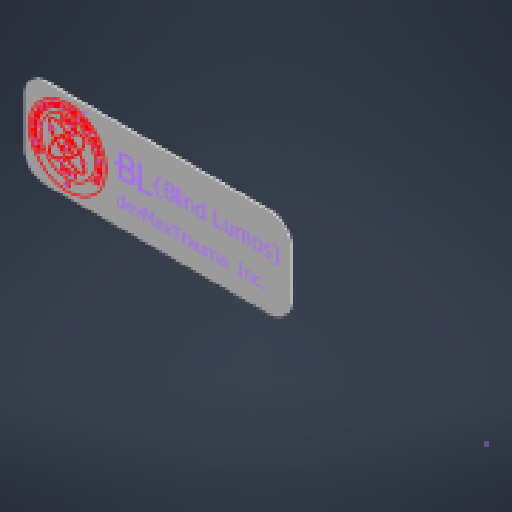
# Autodesk Inventor part: hanabi plate
Saved by Autodesk Inventor 2025.1 (Build 291241020, 241B)
## iProperties
Created: 2024-09-23
Part Number: hanabi plate
Material: Generic
Document SubType Name: Modeling
Designer: techn
Density: 1 g/cm^3
Appearance: Default
Author: techn
Autodesk Inventor part; units mm, degrees
ref_plane "YZ Plane" through (0, 0, 0) normal (1, 0, 0) x (0, 1, 0)
ref_plane "XZ Plane" through (0, 0, 0) normal (0, 1, 0) x (-1, 0, 0)
ref_plane "XY Plane" through (0, 0, 0) normal (0, 0, 1) x (1, 0, 0)
sketch "Sketch1" plane through (0, 0, 0) normal (0, 0, 1) x (1, 0, 0)
  line L0 (3, 0) -> (447, 0)
  line L1 (450, 3) -> (450, 147)
  line L2 (447, 150) -> (3, 150)
  line L3 (0, 147) -> (0, 3)
  arc A0 (3, 150) -> (0, 147) centre (3, 147) ccw
  arc A1 (450, 147) -> (447, 150) centre (447, 147) ccw
  arc A2 (447, 0) -> (450, 3) centre (447, 3) ccw
  arc A3 (0, 3) -> (3, 0) centre (3, 3) ccw
  point P0 (0, 0)
  point P1 (0, 150)
  point P2 (450, 150)
  point P3 (450, 0)
  point P4 (0, 0)
  dimension "d0" = 450
  dimension "d1" = 150
  dimension "d6" = 3
  constraints: 10 point on line, 8 end point, 8 point on circle, 8 tangent, 4 centre point, 3 equal radius, 2 parallel, 1 horizontal, 1 perpendicular
  measures "d0" distance of point (0, 150) point (450, 150)
  measures "d1" distance of point (450, 150) point (450, 0)
  measures "d6" radius of A0
extrude "Extrusion1" add sketch "Sketch1" along normal blind 3
sketch "Sketch2" plane through (0, 0, 3) normal (0, 0, 1) x (1, 0, 0)
  circle A0 centre (74.3304, 73.386) radius 64.4941
  circle A1 centre (74.1358, 19.1374) radius 3.759
  circle A2 centre (74.3304, 73.386) radius 46.1652
  arc A3 (60.0832, 47.8007) -> (66.8292, 50.9644) centre (63.3353, 49.6403) ccw
  arc A4 (102.5659, 60.1821) -> (99.6639, 66.6182) centre (100.186, 62.9813) ccw
  arc A5 (80.1151, 97.5331) -> (86.506, 100.628) centre (82.7963, 100.1425) ccw
  arc A6 (44.8092, 88.9664) -> (47.8294, 82.593) centre (47.2318, 86.2121) ccw
  line L0 (73.0471, 70.515) -> (72.9845, 77.892)
  line L1 (72.9845, 77.892) -> (69.4651, 77.9045)
  line L2 (69.4651, 77.9045) -> (69.5403, 70.4023)
  line L3 (69.5403, 70.4023) -> (62.2134, 70.4148)
  line L4 (62.2134, 70.4148) -> (62.2385, 67.2712)
  line L5 (62.2385, 67.2712) -> (84.0562, 67.2712)
  line L6 (84.0562, 67.2712) -> (84.0562, 70.3898)
  line L7 (84.0562, 70.3898) -> (73.0471, 70.515)
  line L8 (81.7131, 85.3553) -> (64.4794, 85.3954)
  line L9 (64.4794, 85.3954) -> (64.4794, 82.4296)
  line L10 (64.4794, 82.4296) -> (77.8656, 82.4096)
  arc A7 (80.1926, 72.9483) -> (81.7131, 85.3553) centre (16.1968, 87.088) ccw
  arc A8 (76.6977, 73.1086) -> (77.8656, 82.4096) centre (28.8399, 83.8415) ccw
  line L11 (76.6977, 73.1086) -> (80.1926, 72.9483)
  line L12 (22.8218, 44.3119) -> (29.3747, 47.7587)
  line L13 (29.3747, 47.7587) -> (28.6132, 49.3017)
  line L14 (28.6132, 49.3017) -> (25.0462, 47.5182)
  line L15 (25.0462, 47.5182) -> (27.6313, 51.3056)
  line L16 (27.6313, 51.3056) -> (26.8297, 52.8286)
  line L17 (26.8297, 52.8286) -> (20.1165, 49.4821)
  line L18 (20.1165, 49.4821) -> (20.9582, 47.8188)
  line L19 (20.9582, 47.8188) -> (24.3248, 49.5221)
  line L20 (24.3248, 49.5221) -> (21.9, 45.895)
  line L21 (21.9, 45.895) -> (22.8218, 44.3119)
  arc A9 (20.5574, 56.2553) -> (21.4191, 53.8706) centre (21.1012, 55.1038) ccw
  arc A10 (23.0824, 54.552) -> (22.2407, 56.7763) centre (22.685, 55.673) ccw
  arc A11 (21.4191, 53.8706) -> (23.0824, 54.552) centre (20.078, 59.5153) ccw
  arc A12 (24.3636, 53.0797) -> (21.518, 58.5304) centre (22.6001, 55.6272) ccw
  arc A13 (22.1192, 52.1379) -> (24.3636, 53.0797) centre (20.1363, 60.0082) ccw
  line L22 (19.9149, 57.9493) -> (20.5574, 56.2553)
  line L23 (21.518, 58.5304) -> (22.2407, 56.7763)
  line L24 (15.5802, 64.2799) -> (16.032, 62.5112)
  line L25 (16.032, 62.5112) -> (18.4166, 62.9721)
  line L26 (18.4166, 62.9721) -> (18.9176, 61.0684)
  line L27 (18.9176, 61.0684) -> (16.4127, 60.6075)
  line L28 (16.4127, 60.6075) -> (16.8536, 58.7639)
  line L29 (16.8536, 58.7639) -> (24.0877, 60.2668)
  line L30 (24.0877, 60.2668) -> (23.727, 62.0503)
  line L31 (23.727, 62.0503) -> (20.6811, 61.4892)
  line L32 (20.6811, 61.4892) -> (20.3604, 63.3729)
  line L33 (20.3604, 63.3729) -> (23.2661, 64.0342)
  line L34 (23.2661, 64.0342) -> (22.8854, 65.8177)
  line L35 (22.8854, 65.8177) -> (15.5802, 64.2799)
  line L36 (14.9282, 71.5177) -> (15.4291, 66.3877)
  line L37 (15.4291, 66.3877) -> (22.8036, 66.9087)
  line L38 (22.8036, 66.9087) -> (22.3627, 72.3593)
  line L39 (22.3627, 72.3593) -> (20.5191, 72.2191)
  line L40 (20.5191, 72.2191) -> (20.8397, 68.6721)
  line L41 (20.8397, 68.6721) -> (19.6374, 68.632)
  line L42 (19.6374, 68.632) -> (19.4169, 71.5979)
  line L43 (19.4169, 71.5979) -> (17.6334, 71.4776)
  line L44 (17.6334, 71.4776) -> (17.8739, 68.4717)
  line L45 (17.8739, 68.4717) -> (16.9922, 68.4317)
  line L46 (16.9922, 68.4317) -> (16.6716, 71.678)
  line L47 (16.6716, 71.678) -> (14.9282, 71.5177)
  ellipse E0 centre (18.7456, 76.2269) end of major axis (16.6515, 76.3071) minor radius 1.427
  ellipse E1 centre (18.7256, 76.1868) end of major axis (14.828, 76.3872) minor radius 3.5212
  line L48 (15.4067, 81.6515) -> (15.7474, 83.3549)
  line L49 (15.7474, 83.3549) -> (19.8153, 84.6975)
  line L50 (19.8153, 84.6975) -> (16.088, 85.4389)
  line L51 (16.088, 85.4389) -> (16.2884, 87.1623)
  line L52 (16.2884, 87.1623) -> (23.7029, 85.8598)
  line L53 (23.7029, 85.8598) -> (23.5025, 84.2566)
  line L54 (23.5025, 84.2566) -> (19.0338, 82.8138)
  line L55 (19.0338, 82.8138) -> (23.0216, 82.0723)
  line L56 (23.0216, 82.0723) -> (22.7811, 80.2488)
  line L57 (22.7811, 80.2488) -> (15.4067, 81.6515)
  line L58 (19.7752, 97.1418) -> (17.8715, 92.2723)
  line L59 (17.8715, 92.2723) -> (24.745, 89.7073)
  line L60 (24.745, 89.7073) -> (26.6487, 94.6169)
  line L61 (26.6487, 94.6169) -> (25.1658, 95.2581)
  line L62 (25.1658, 95.2581) -> (23.9434, 92.0719)
  line L63 (23.9434, 92.0719) -> (22.6609, 92.5529)
  line L64 (22.6609, 92.5529) -> (23.743, 95.3183)
  line L65 (23.743, 95.3183) -> (22.1599, 95.9395)
  line L66 (22.1599, 95.9395) -> (21.0778, 93.0939)
  line L67 (21.0778, 93.0939) -> (20.0758, 93.4747)
  line L68 (20.0758, 93.4747) -> (21.2782, 96.5206)
  line L69 (21.2782, 96.5206) -> (19.7752, 97.1418)
  line L70 (21.3984, 100.3882) -> (20.3764, 98.765)
  line L71 (20.3764, 98.765) -> (27.0094, 95.3383)
  line L72 (27.0094, 95.3383) -> (29.3339, 99.9273)
  line L73 (29.3339, 99.9273) -> (27.7909, 100.6888)
  line L74 (27.7909, 100.6888) -> (26.3681, 97.8833)
  line L75 (26.3681, 97.8833) -> (21.3984, 100.3882)
  line L76 (29.7347, 100.3882) -> (32.7206, 104.917)
  line L77 (32.7206, 104.917) -> (31.2577, 105.9591)
  line L78 (31.2577, 105.9591) -> (29.2939, 103.0334)
  line L79 (29.2939, 103.0334) -> (28.2518, 103.6746)
  line L80 (28.2518, 103.6746) -> (29.9752, 106.2998)
  line L81 (29.9752, 106.2998) -> (28.5725, 107.1815)
  line L82 (28.5725, 107.1815) -> (26.789, 104.6365)
  line L83 (26.789, 104.6365) -> (25.9674, 105.1976)
  line L84 (25.9674, 105.1976) -> (27.9312, 107.943)
  line L85 (27.9312, 107.943) -> (26.4884, 108.9249)
  line L86 (26.4884, 108.9249) -> (23.4625, 104.6165)
  line L87 (23.4625, 104.6165) -> (29.7347, 100.3882)
  line L88 (32.42, 111.7103) -> (33.6223, 113.073)
  line L89 (34.8848, 112.0109) -> (33.6223, 110.6082)
  arc A14 (30.5404, 107.4866) -> (34.8848, 112.0109) centre (32.7697, 109.6939) ccw
  arc A15 (33.6223, 113.073) -> (29.2378, 108.8017) centre (31.6861, 110.6746) ccw
  arc A16 (29.2378, 108.8017) -> (30.5404, 107.4866) centre (52.0371, 130.0812) ccw
  arc A17 (32.42, 111.7103) -> (30.7157, 109.9915) centre (31.6602, 110.7594) ccw
  arc A18 (32.0912, 108.6533) -> (33.6223, 110.6082) centre (32.9043, 109.5936) ccw
  arc A19 (30.7157, 109.9915) -> (32.0912, 108.6533) centre (34.3325, 112.3331) ccw
  line L90 (36.7024, 119.6663) -> (37.8847, 118.4238)
  line L91 (37.8847, 118.4238) -> (36.502, 117.1413)
  line L92 (36.502, 117.1413) -> (40.2293, 112.913)
  line L93 (40.2293, 112.913) -> (38.8666, 111.6506)
  line L94 (38.8666, 111.6506) -> (35.0391, 115.8588)
  line L95 (35.0391, 115.8588) -> (33.5362, 114.5563)
  line L96 (33.5362, 114.5563) -> (32.3739, 115.8588)
  line L97 (32.3739, 115.8588) -> (36.7024, 119.6663)
  line L98 (38.0651, 120.7283) -> (42.2533, 114.6565)
  line L99 (42.2533, 114.6565) -> (43.636, 115.6584)
  line L100 (43.636, 115.6584) -> (42.2332, 117.8026)
  line L101 (42.2332, 117.8026) -> (43.5558, 118.7044)
  line L102 (38.0651, 120.7283) -> (41.2914, 122.9527)
  line L103 (45.4555, 116.9645) -> (47.0226, 118.023)
  line L104 (47.0226, 118.023) -> (46.7462, 118.4132)
  line L105 (46.7462, 118.4132) -> (46.3989, 118.4328)
  line L106 (46.3989, 118.4328) -> (45.4247, 119.8307)
  line L107 (45.4555, 116.9645) -> (44.134, 118.5977)
  arc A20 (44.134, 118.5977) -> (43.5558, 118.7044) centre (43.8033, 118.4259) ccw
  arc A21 (45.4247, 119.8307) -> (44.2896, 120.3317) centre (44.5184, 119.3138) ccw
  arc A22 (44.2896, 120.3317) -> (41.2914, 122.9527) centre (42.2418, 121.0145) ccw
  line L108 (40.5088, 120.363) -> (41.2524, 119.2828)
  line L109 (41.2524, 119.2828) -> (42.5988, 120.2221)
  line L110 (41.8787, 121.3102) -> (40.5088, 120.363)
  arc A23 (42.5988, 120.2221) -> (41.8787, 121.3102) centre (42.1607, 120.7145) ccw
  ellipse E2 centre (48.8933, 123.1148) end of major axis (47.8713, 124.9484) minor radius 1.3869
  ellipse E3 centre (48.9333, 123.1048) end of major axis (47.0296, 126.4514) minor radius 3.3442
  line L111 (51.8591, 128.6156) -> (53.5824, 129.1767)
  line L112 (53.5824, 129.1767) -> (56.949, 126.3311)
  line L113 (56.949, 126.3311) -> (55.6465, 130.0384)
  line L114 (55.6465, 130.0384) -> (57.2296, 130.4392)
  line L115 (57.2296, 130.4392) -> (59.7144, 123.5256)
  line L116 (59.7144, 123.5256) -> (58.0913, 122.9645)
  line L117 (58.0913, 122.9645) -> (54.6846, 126.0305)
  line L118 (54.6846, 126.0305) -> (55.927, 122.2231)
  line L119 (55.927, 122.2231) -> (54.2838, 121.682)
  line L120 (54.2838, 121.682) -> (51.8591, 128.6156)
  line L121 (59.1333, 130.9602) -> (60.9769, 131.381)
  line L122 (60.9769, 131.381) -> (62.7003, 124.2671)
  line L123 (62.7003, 124.2671) -> (60.9969, 123.8262)
  line L124 (60.9969, 123.8262) -> (59.1333, 130.9602)
  arc A24 (65.2629, 127.4613) -> (67.7678, 127.9022) centre (66.5191, 127.6602) ccw
  arc A25 (67.4947, 129.7232) -> (65.0149, 129.2974) centre (66.2808, 129.3592) ccw
  arc A26 (69.2357, 129.9737) -> (63.1362, 128.9091) centre (66.2187, 129.2539) ccw
  arc A27 (63.4994, 127.1432) -> (69.4235, 128.0199) centre (66.453, 127.6388) ccw
  arc A28 (63.1362, 128.9091) -> (63.4994, 127.1432) centre (67.9042, 128.9695) ccw
  arc A29 (65.0149, 129.2974) -> (65.2629, 127.4613) centre (79.0489, 130.2581) ccw
  line L125 (67.4947, 129.7232) -> (69.2357, 129.9737)
  line L126 (67.7678, 127.9022) -> (69.4235, 128.0199)
  line L127 (73.8923, 132.8018) -> (76.2469, 132.7391)
  line L128 (76.2469, 132.7391) -> (76.9608, 128.5434)
  line L129 (76.9608, 128.5434) -> (78.2132, 132.5638)
  line L130 (78.2132, 132.5638) -> (80.4802, 132.426)
  line L131 (80.4802, 132.426) -> (80.0543, 125.1994)
  line L132 (80.0543, 125.1994) -> (78.4136, 125.2745)
  line L133 (78.4136, 125.2745) -> (78.6015, 128.08)
  line L134 (78.6015, 128.08) -> (77.612, 125.3998)
  line L135 (77.612, 125.3998) -> (75.9588, 125.4123)
  line L136 (75.9588, 125.4123) -> (75.3576, 128.5309)
  line L137 (75.3576, 128.5309) -> (75.1322, 125.4874)
  line L138 (75.1322, 125.4874) -> (73.4414, 125.6002)
  line L139 (73.4414, 125.6002) -> (73.8923, 132.8018)
  line L140 (81.0939, 125.0491) -> (86.279, 123.997)
  line L141 (86.279, 123.997) -> (86.6046, 125.5751)
  line L142 (86.6046, 125.5751) -> (83.0978, 126.2264)
  line L143 (83.0978, 126.2264) -> (83.3984, 127.6041)
  line L144 (83.3984, 127.6041) -> (86.5044, 127.053)
  line L145 (86.5044, 127.053) -> (86.7925, 128.5935)
  line L146 (86.7925, 128.5935) -> (83.7365, 129.1571)
  line L147 (83.7365, 129.1571) -> (83.8994, 130.2342)
  line L148 (83.8994, 130.2342) -> (87.1682, 129.5579)
  line L149 (87.1682, 129.5579) -> (87.5064, 131.1235)
  line L150 (87.5064, 131.1235) -> (82.4841, 132.163)
  line L151 (82.4841, 132.163) -> (81.0939, 125.0491)
  line L152 (89.2849, 130.6976) -> (90.9757, 130.1841)
  line L153 (90.9757, 130.1841) -> (88.9092, 123.208)
  line L154 (88.9092, 123.208) -> (87.1682, 123.6589)
  line L155 (87.1682, 123.6589) -> (89.2849, 130.6976)
  line L156 (90.9953, 125.1721) -> (92.4983, 124.611)
  line L157 (95.3038, 126.0338) -> (96.8869, 125.3725)
  arc A30 (90.9953, 125.1721) -> (96.1053, 122.8275) centre (93.6122, 124.1346) ccw
  arc A31 (96.8869, 125.3725) -> (91.857, 127.4967) centre (94.3068, 126.2803) ccw
  arc A32 (91.857, 127.4967) -> (93.4401, 124.6311) centre (94.2672, 126.9581) ccw
  arc A33 (96.1053, 122.8275) -> (94.9631, 125.6731) centre (93.9846, 123.6283) ccw
  arc A34 (95.3038, 126.0338) -> (93.5403, 127.176) centre (94.2317, 126.311) ccw
  arc A35 (93.5403, 127.176) -> (93.8409, 126.4146) centre (93.9888, 126.913) ccw
  arc A36 (93.8409, 126.4146) -> (94.9631, 125.6731) centre (103.26, 139.4505) ccw
  line L158 (93.4401, 124.6311) -> (94.4822, 123.8896)
  arc A37 (94.2417, 123.048) -> (94.4822, 123.8896) centre (94.0571, 123.5559) ccw
  arc A38 (92.8059, 123.2884) -> (94.2417, 123.048) centre (93.781, 124.7043) ccw
  arc A39 (92.4983, 124.611) -> (92.8059, 123.2884) centre (93.1362, 124.0623) ccw
  line L159 (100.1226, 124.5633) -> (97.4935, 119.6577)
  line L160 (97.4935, 119.6577) -> (99.0966, 118.7279)
  line L161 (99.0966, 118.7279) -> (101.854, 123.7297)
  line L162 (101.854, 123.7297) -> (103.5854, 122.7999)
  line L163 (103.5854, 122.7999) -> (104.419, 124.1786)
  line L164 (104.419, 124.1786) -> (99.3852, 127.0322)
  line L165 (99.3852, 127.0322) -> (98.4554, 125.5893)
  line L166 (98.4554, 125.5893) -> (100.1226, 124.5633)
  line L167 (101.5053, 117.4294) -> (105.7536, 123.4211)
  line L168 (105.7536, 123.4211) -> (109.9218, 120.4353)
  line L169 (109.9218, 120.4353) -> (108.9399, 119.0125)
  line L170 (108.9399, 119.0125) -> (106.1945, 120.8962)
  line L171 (106.1945, 120.8962) -> (105.6935, 120.1948)
  line L172 (105.6935, 120.1948) -> (108.2185, 118.3512)
  line L173 (108.2185, 118.3512) -> (107.2566, 117.0486)
  line L174 (107.2566, 117.0486) -> (104.6715, 118.752)
  line L175 (104.6715, 118.752) -> (103.9501, 117.73)
  line L176 (103.9501, 117.73) -> (106.7957, 115.6659)
  line L177 (106.7957, 115.6659) -> (105.7136, 114.2832)
  line L178 (105.7136, 114.2832) -> (101.5053, 117.4294)
  line L179 (111.3646, 119.1928) -> (106.3147, 113.7422)
  line L180 (106.3147, 113.7422) -> (107.6774, 112.5498)
  line L181 (107.6774, 112.5498) -> (109.501, 114.5037)
  line L182 (109.501, 114.5037) -> (110.7033, 113.5017)
  line L183 (111.3646, 119.1928) -> (114.1864, 116.6281)
  line L184 (112.7774, 115.5656) -> (111.6374, 116.6713)
  line L185 (111.6374, 116.6713) -> (110.8351, 115.7515)
  line L186 (110.8351, 115.7515) -> (111.8772, 114.7094)
  line L187 (110.6791, 112.9268) -> (109.2764, 111.2235)
  line L188 (109.2764, 111.2235) -> (110.7621, 109.8192)
  line L189 (110.7621, 109.8192) -> (111.13, 110.1949)
  line L190 (111.13, 110.1949) -> (111.0282, 110.5706)
  line L191 (111.0282, 110.5706) -> (112.2729, 111.9014)
  arc A40 (110.6791, 112.9268) -> (110.7033, 113.5017) centre (110.3532, 113.2285) ccw
  arc A41 (112.2729, 111.9014) -> (112.4178, 113.0193) centre (111.1593, 112.6141) ccw
  arc A42 (111.8772, 114.7094) -> (112.7774, 115.5656) centre (112.2379, 115.2315) ccw
  arc A43 (112.4178, 113.0193) -> (114.1864, 116.6281) centre (112.538, 115.1982) ccw
  line L192 (113.3248, 107.0457) -> (119.0961, 111.4343)
  line L193 (119.0961, 111.4343) -> (120.2784, 109.9514)
  line L194 (120.2784, 109.9514) -> (118.2144, 108.4284)
  line L195 (118.2144, 108.4284) -> (119.4368, 106.8052)
  line L196 (119.4368, 106.8052) -> (121.4607, 108.3081)
  line L197 (121.4607, 108.3081) -> (122.623, 106.8052)
  line L198 (122.623, 106.8052) -> (116.6714, 102.3966)
  line L199 (116.6714, 102.3966) -> (115.5893, 103.8594)
  line L200 (115.5893, 103.8594) -> (117.9739, 105.683)
  line L201 (117.9739, 105.683) -> (116.8116, 107.3262)
  line L202 (116.8116, 107.3262) -> (114.3268, 105.5227)
  line L203 (114.3268, 105.5227) -> (113.3248, 107.0457)
  line L204 (117.3727, 101.3545) -> (123.5448, 105.162)
  line L205 (123.5448, 105.162) -> (124.5468, 103.5388)
  line L206 (124.5468, 103.5388) -> (118.2745, 99.7314)
  line L207 (118.2745, 99.7314) -> (117.3727, 101.3545)
  line L208 (123.2155, 95.6967) -> (122.5542, 96.8791)
  line L209 (122.5542, 96.8791) -> (124.0572, 97.6606)
  line L210 (124.0572, 97.6606) -> (125.3998, 94.9553)
  line L211 (125.3998, 94.9553) -> (121.6926, 93.0315)
  line L212 (121.6926, 93.0315) -> (120.9912, 94.4142)
  line L213 (120.9912, 94.4142) -> (121.3118, 94.6948)
  arc A44 (121.9731, 98.0213) -> (123.2155, 95.6967) centre (122.9571, 97.0529) ccw
  arc A45 (124.0271, 99.131) -> (121.9731, 98.0213) centre (124.5431, 95.72) ccw
  arc A46 (125.2044, 96.7012) -> (124.0271, 99.131) centre (124.3539, 97.7892) ccw
  line L214 (125.2044, 96.7012) -> (125.981, 95.0354)
  arc A47 (125.981, 95.0354) -> (122.8498, 100.7216) centre (124.119, 97.7153) ccw
  arc A48 (122.8498, 100.7216) -> (120.1946, 98.8178) centre (124.2192, 96.0082) ccw
  arc A49 (120.1946, 98.8178) -> (121.3118, 94.6948) centre (122.701, 97.2841) ccw
  line L215 (122.0117, 92.1357) -> (128.8731, 94.348)
  line L216 (128.8731, 94.348) -> (129.4823, 92.7128)
  line L217 (129.4823, 92.7128) -> (126.9494, 91.8792)
  line L218 (126.9494, 91.8792) -> (127.7509, 89.6989)
  line L219 (127.7509, 89.6989) -> (130.0595, 90.5005)
  line L220 (130.0595, 90.5005) -> (130.6045, 88.9615)
  line L221 (130.6045, 88.9615) -> (123.6469, 86.7492)
  line L222 (123.6469, 86.7492) -> (123.2622, 88.3523)
  line L223 (123.2622, 88.3523) -> (126.0837, 89.3462)
  line L224 (126.0837, 89.3462) -> (125.5386, 91.3662)
  line L225 (125.5386, 91.3662) -> (122.4606, 90.4684)
  line L226 (122.4606, 90.4684) -> (122.0117, 92.1357)
  line L227 (127.1227, 83.2797) -> (127.2229, 81.6766)
  line L228 (129.7879, 79.7628) -> (129.9758, 78.1847)
  arc A50 (127.1227, 83.2797) -> (126.8547, 77.5109) centre (127.4108, 80.3757) ccw
  arc A51 (129.9758, 78.1847) -> (130.081, 83.6629) centre (129.6354, 80.9314) ccw
  arc A52 (130.081, 83.6629) -> (127.8241, 81.7918) centre (129.9946, 81.4705) ccw
  arc A53 (127.2229, 81.6766) -> (126.2836, 80.5769) centre (127.3612, 80.6074) ccw
  arc A54 (126.2836, 80.5769) -> (126.747, 79.4622) centre (127.8549, 80.5765) ccw
  arc A55 (126.747, 79.4622) -> (127.5486, 79.7252) centre (127.0889, 79.7732) ccw
  arc A56 (127.8241, 81.7918) -> (127.5486, 79.7252) centre (778.3659, -5.9988) ccw
  arc A57 (129.7879, 79.7628) -> (130.2163, 81.8419) centre (129.4879, 80.9083) ccw
  arc A58 (130.2163, 81.8419) -> (129.5775, 81.5037) centre (130.0077, 81.4634) ccw
  arc A59 (129.1642, 78.8861) -> (129.5775, 81.5037) centre (45.9299, 93.3698) ccw
  arc A60 (126.8547, 77.5109) -> (129.1642, 78.8861) centre (127.0095, 79.8778) ccw
  ellipse E4 centre (128.9018, 73.4046) end of major axis (126.7676, 73.4246) minor radius 1.3445 (129.8941, 72.2086) -> (128.0696, 72.1712) ccw
  ellipse E5 centre (128.9118, 73.4747) end of major axis (125.0443, 73.4847) minor radius 3.1768 (129.9327, 70.4097) -> (128.0695, 70.3749) ccw
  line L229 (128.0702, 70.3786) -> (128.0695, 70.3749)
  line L230 (129.8941, 72.2086) -> (129.9327, 70.4097)
  line L231 (128.0702, 72.1711) -> (128.0702, 70.3786)
  line L232 (128.0696, 72.1712) -> (128.0702, 72.1711)
  line L233 (125.2047, 69.6146) -> (132.4362, 68.5719)
  line L234 (132.4362, 68.5719) -> (132.2176, 66.7556)
  line L235 (132.2176, 66.7556) -> (129.5436, 67.0415)
  line L236 (129.5436, 67.0415) -> (129.325, 65.0402)
  line L237 (129.325, 65.0402) -> (131.9653, 64.7039)
  line L238 (131.9653, 64.7039) -> (131.6962, 62.9212)
  line L239 (131.6962, 62.9212) -> (124.2629, 63.9303)
  line L240 (124.2629, 63.9303) -> (124.5488, 65.797)
  line L241 (124.5488, 65.797) -> (127.6937, 65.3766)
  line L242 (127.6937, 65.3766) -> (127.9291, 67.2938)
  line L243 (127.9291, 67.2938) -> (124.8683, 67.6469)
  line L244 (124.8683, 67.6469) -> (125.2047, 69.6146)
  ellipse E6 centre (126.872, 58.825) end of major axis (124.9296, 59.4724) minor radius 1.5069
  ellipse E7 centre (126.8552, 58.7829) end of major axis (123.2647, 60.2292) minor radius 3.2341
  ellipse E8 centre (124.2064, 51.5934) end of major axis (122.3397, 52.4763) minor radius 1.4344
  ellipse E9 centre (124.2989, 51.5682) end of major axis (120.9606, 53.5022) minor radius 3.3298
  line L245 (119.6993, 46.8088) -> (118.0344, 44.1012)
  line L246 (118.0344, 44.1012) -> (116.4703, 45.0598)
  line L247 (116.4703, 45.0598) -> (119.0939, 49.3483)
  line L248 (119.0939, 49.3483) -> (125.5518, 45.6484)
  line L249 (125.5518, 45.6484) -> (124.5092, 44.0003)
  line L250 (124.5092, 44.0003) -> (119.6993, 46.8088)
  arc A61 (66.937, 40.1205) -> (61.7975, 40.0936) centre (64.3667, 40.2125) ccw
  arc A62 (65.6866, 40.3787) -> (62.9748, 40.0633) centre (64.3345, 40.1883) ccw
  arc A63 (65.119, 39.1384) -> (65.6866, 40.3787) centre (64.3203, 40.2539) ccw
  line L251 (61.7975, 40.0936) -> (62.9748, 40.0633)
  line L252 (65.119, 39.1384) -> (61.7256, 35.7606)
  line L253 (61.7256, 35.7606) -> (61.7256, 34.6674)
  line L254 (61.7256, 34.6674) -> (66.8718, 34.6674)
  line L255 (66.8718, 34.6674) -> (66.8718, 35.8783)
  line L256 (66.8718, 35.8783) -> (63.4242, 35.8951)
  line L257 (63.4242, 35.8951) -> (66.2664, 38.6364)
  arc A64 (66.2664, 38.6364) -> (66.937, 40.1205) centre (64.8521, 40.169) ccw
  arc A65 (72.6467, 40.4747) -> (69.7982, 40.4852) centre (71.2209, 40.0648) ccw
  arc A66 (73.971, 40.296) -> (68.3687, 40.4432) centre (71.1599, 39.9911) ccw
  arc A67 (69.8087, 36.7223) -> (72.7413, 37.0376) centre (71.2359, 37.243) ccw
  arc A68 (68.3582, 36.8905) -> (74.0236, 37.2689) centre (71.1847, 37.173) ccw
  line L258 (68.3687, 40.4432) -> (68.3582, 36.8905)
  line L259 (69.8087, 36.7223) -> (69.7982, 40.4852)
  line L260 (72.6467, 40.4747) -> (72.7413, 37.0376)
  line L261 (74.0236, 37.2689) -> (73.971, 40.296)
  line L262 (76.2507, 42.6737) -> (78.9247, 42.6737)
  line L263 (78.9247, 42.6737) -> (78.9247, 34.7358)
  line L264 (78.9247, 34.7358) -> (77.6742, 34.7359)
  line L265 (77.6742, 34.7359) -> (77.6633, 41.6142)
  line L266 (77.6633, 41.6142) -> (76.2528, 41.6191)
  line L267 (76.2528, 41.6191) -> (76.2507, 42.6737)
  arc A69 (86.5806, 40.4747) -> (83.7321, 40.4852) centre (85.1548, 40.0648) ccw
  arc A70 (87.905, 40.296) -> (82.3026, 40.4432) centre (85.0938, 39.9911) ccw
  arc A71 (83.7426, 36.7223) -> (86.6752, 37.0376) centre (85.1699, 37.243) ccw
  arc A72 (82.2921, 36.8905) -> (87.9575, 37.2689) centre (85.1186, 37.173) ccw
  line L268 (82.3026, 40.4432) -> (82.2921, 36.8905)
  line L269 (83.7426, 36.7223) -> (83.7321, 40.4852)
  line L270 (86.5806, 40.4747) -> (86.6752, 37.0376)
  line L271 (87.9575, 37.2689) -> (87.905, 40.296)
  line L272 (62.4142, 114.1934) -> (65.0882, 114.1934)
  line L273 (65.0882, 114.1934) -> (65.0882, 106.2555)
  line L274 (65.0882, 106.2555) -> (63.8378, 106.2556)
  line L275 (63.8378, 106.2556) -> (63.8269, 113.1339)
  line L276 (63.8269, 113.1339) -> (62.4164, 113.1388)
  line L277 (62.4164, 113.1388) -> (62.4142, 114.1934)
  circle A73 centre (71.262, 111.5976) radius 1.6109
  arc A74 (73.6726, 110.1228) -> (71.3999, 108.7522) centre (71.2213, 111.6179) ccw
  line L278 (69.6746, 106.3394) -> (71.2772, 106.3522)
  line L279 (71.2772, 106.3522) -> (73.6726, 110.1228)
  line L280 (71.3999, 108.7522) -> (69.6746, 106.3394)
  line L281 (77.0239, 111.4154) -> (77.3696, 113.0687)
  line L282 (77.3696, 113.0687) -> (80.2402, 113.0837)
  line L283 (80.2402, 113.0837) -> (80.2214, 114.2579)
  line L284 (80.2214, 114.2579) -> (76.4359, 114.2297)
  line L285 (76.4359, 114.2297) -> (75.6927, 110.168)
  arc A75 (76.506, 108.7627) -> (76.7496, 109.8583) centre (78.1408, 108.9741) ccw
  arc A76 (75.369, 108.7627) -> (77.0239, 111.4154) centre (78.184, 108.8491) ccw
  line L286 (76.7496, 109.8583) -> (75.6927, 110.168)
  line L287 (76.506, 108.7627) -> (75.369, 108.7627)
  arc A77 (87.675, 111.5415) -> (82.5356, 111.5146) centre (85.1047, 111.6335) ccw
  arc A78 (86.4246, 111.7997) -> (83.7128, 111.4843) centre (85.0725, 111.6093) ccw
  arc A79 (85.857, 110.5594) -> (86.4246, 111.7997) centre (85.0583, 111.6749) ccw
  line L288 (82.5356, 111.5146) -> (83.7128, 111.4843)
  line L289 (85.857, 110.5594) -> (82.4637, 107.1816)
  line L290 (82.4637, 107.1816) -> (82.4637, 106.0884)
  line L291 (82.4637, 106.0884) -> (87.6098, 106.0884)
  line L292 (87.6098, 106.0884) -> (87.6098, 107.2993)
  line L293 (87.6098, 107.2993) -> (84.1622, 107.3161)
  line L294 (84.1622, 107.3161) -> (87.0044, 110.0574)
  arc A80 (87.0044, 110.0574) -> (87.675, 111.5415) centre (85.5902, 111.59) ccw
  ellipse E10 centre (73.5541, 74.9499) end of major axis (101.9248, 101.7351) minor radius 15.3231 (66.8292, 50.9644) -> (73.5687, 55.2013) ccw
  ellipse E11 centre (73.5541, 74.9499) end of major axis (45.2119, 101.6505) minor radius 15.3224 (47.8294, 82.593) -> (52.9403, 74.9433) ccw
  ellipse E12 centre (73.5541, 74.9499) end of major axis (46.1113, 101.2061) minor radius 14.1544 (48.9856, 82.9904) -> (53.7136, 75.9402) ccw
  ellipse E13 centre (73.5541, 74.9499) end of major axis (45.9927, 49.2842) minor radius 14.2819 (66.2633, 51.9614) -> (72.6054, 55.8854) ccw
  arc A81 (48.9856, 82.9904) -> (45.8108, 89.5938) centre (47.2318, 86.2121) ccw
  arc A82 (66.2633, 51.9614) -> (59.6702, 48.9143) centre (63.3353, 49.6403) ccw
  ellipse E14 centre (73.5541, 74.9499) end of major axis (101.9248, 101.7351) minor radius 15.3231 (79.4501, 98.4689) -> (73.5395, 94.6985) ccw
  ellipse E15 centre (73.5541, 74.9499) end of major axis (45.9927, 49.2842) minor radius 14.2819 (80.1151, 97.5331) -> (74.5028, 94.0144) ccw
  arc A83 (86.1677, 101.7647) -> (79.4501, 98.4689) centre (82.7963, 100.1425) ccw
  ellipse E16 centre (73.5541, 74.9499) end of major axis (46.1113, 101.2061) minor radius 14.1544 (98.501, 66.2464) -> (93.3946, 73.9596) ccw
  ellipse E17 centre (73.5541, 74.9499) end of major axis (45.2119, 101.6505) minor radius 15.3224 (99.6639, 66.6182) -> (94.1679, 74.9565) ccw
  arc A84 (98.501, 66.2464) -> (101.5578, 59.5728) centre (100.186, 62.9813) ccw
  ellipse E18 centre (73.5541, 74.9499) end of major axis (46.1113, 101.2061) minor radius 14.1544 (54.3116, 75.1605) -> (73.5195, 56.5237) ccw
  ellipse E19 centre (73.5541, 74.9499) end of major axis (45.2119, 101.6505) minor radius 15.3224 (53.538, 74.1705) -> (72.6054, 55.8854) ccw
  ellipse E20 centre (73.5541, 74.9499) end of major axis (101.9248, 101.7351) minor radius 15.3231 (52.9403, 74.9433) -> (60.0832, 47.8007) ccw
  ellipse E21 centre (73.5541, 74.9499) end of major axis (45.9927, 49.2842) minor radius 14.2819 (53.538, 74.1705) -> (59.6702, 48.9143) ccw
  ellipse E22 centre (73.5541, 74.9499) end of major axis (45.9927, 49.2842) minor radius 14.2819 (73.5195, 56.5237) -> (92.7965, 74.7393) ccw
  ellipse E23 centre (73.5541, 74.9499) end of major axis (46.1113, 101.2061) minor radius 14.1544 (74.4665, 55.8405) -> (101.5578, 59.5728) ccw
  ellipse E24 centre (73.5541, 74.9499) end of major axis (45.2119, 101.6505) minor radius 15.3224 (73.5687, 55.2013) -> (102.5659, 60.1821) ccw
  ellipse E25 centre (73.5541, 74.9499) end of major axis (101.9248, 101.7351) minor radius 15.3231 (74.4665, 55.8405) -> (93.3946, 73.9596) ccw
  ellipse E26 centre (73.5541, 74.9499) end of major axis (101.9248, 101.7351) minor radius 15.3231 (72.6417, 94.0592) -> (53.7136, 75.9402) ccw
  ellipse E27 centre (73.5541, 74.9499) end of major axis (46.1113, 101.2061) minor radius 14.1544 (72.6417, 94.0592) -> (45.8108, 89.5938) ccw
  ellipse E28 centre (73.5541, 74.9499) end of major axis (45.2119, 101.6505) minor radius 15.3224 (73.5395, 94.6985) -> (44.8092, 88.9664) ccw
  ellipse E29 centre (73.5541, 74.9499) end of major axis (45.9927, 49.2842) minor radius 14.2819 (73.5887, 93.3761) -> (54.3116, 75.1605) ccw
  ellipse E30 centre (73.5541, 74.9499) end of major axis (101.9248, 101.7351) minor radius 15.3231 (94.1679, 74.9565) -> (86.1677, 101.7647) ccw
  ellipse E31 centre (73.5541, 74.9499) end of major axis (45.9927, 49.2842) minor radius 14.2819 (93.5702, 75.7292) -> (86.506, 100.628) ccw
  ellipse E32 centre (73.5541, 74.9499) end of major axis (46.1113, 101.2061) minor radius 14.1544 (92.7965, 74.7393) -> (73.5887, 93.3761) ccw
  ellipse E33 centre (73.5541, 74.9499) end of major axis (45.2119, 101.6505) minor radius 15.3224 (93.5702, 75.7292) -> (74.5028, 94.0144) ccw
  arc A85 (19.9149, 57.9493) -> (22.1192, 52.1379) centre (21.0542, 55.0576) ccw
  line L295 (29.9758, 46.7567) -> (31.0379, 45.2538)
  line L296 (31.0379, 45.2538) -> (24.7857, 41.1658)
  line L297 (24.7857, 41.1658) -> (23.7837, 42.7288)
  line L298 (23.7837, 42.7288) -> (29.9758, 46.7567)
  line L299 (156.501, 124.8569) -> (430.6798, 124.8569) construction
  line L300 (430.6798, 124.8569) -> (430.6798, 58.1066) construction
  line L301 (430.6798, 58.1066) -> (156.501, 58.1066) construction
  line L302 (156.501, 58.1066) -> (156.501, 124.8569) construction
  line L303 (220.3273, 107.9931) -> (430.6798, 107.9931) construction
  line L304 (430.6798, 107.9931) -> (430.6798, 74.9704) construction
  line L305 (430.6798, 74.9704) -> (220.3273, 74.9704) construction
  line L306 (220.3273, 74.9704) -> (220.3273, 107.9931) construction
  line L307 (156.501, 51.087) -> (405.9499, 51.087) construction
  line L308 (405.9499, 51.087) -> (405.9499, 29.7742) construction
  line L309 (405.9499, 29.7742) -> (156.501, 29.7742) construction
  line L310 (156.501, 29.7742) -> (156.501, 51.087) construction
  point P0 (156.501, 91.4818)
  point P1 (220.3273, 91.4818)
  constraints: 598 end point, 164 point on circle, 86 centre point, 2 midpoint, 2 vertical alignment, 1 horizontal alignment, 126 other
body "Solid1"
